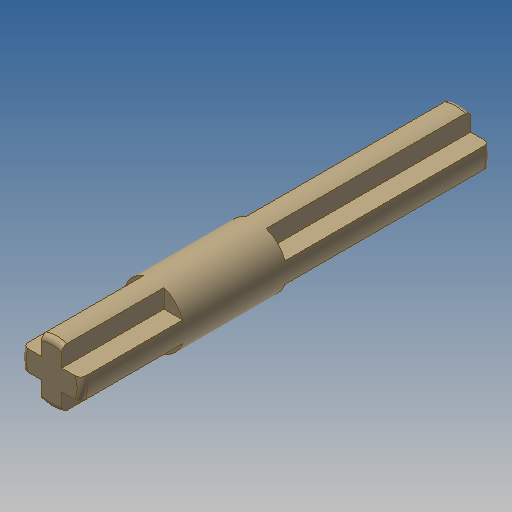
# Autodesk Inventor part: 99008-Tan
Saved by Autodesk Inventor 2022.2 (Build 262287000, 287)
## iProperties
Created: 2014-11-20
Part Number: 99008-Tan
Material: ABS Plastic
Document SubType Name: Modeling
Designer: D. Kohfeld
Mass: 0.471237 g
Surface Area: 5.91487 cm^2
Volume: 0.444563 cm^3
Density: 1.06 g/cm^3
Appearance: Tan
Author: D. Kohfeld
Autodesk Inventor part; units mm, degrees
ref_plane "YZ Plane" through (0, 0, 0) normal (1, 0, 0) x (0, 1, 0)
ref_plane "XZ Plane" through (0, 0, 0) normal (0, 1, 0) x (-1, 0, 0)
ref_plane "XY Plane" through (0, 0, 0) normal (0, 0, 1) x (1, 0, 0)
sketch "Sketch1" plane through (0, 0, 0) normal (0, 0, 1) x (1, 0, 0)
  circle A0 centre (0, 0) radius 2.4
  dimension "d0" = 4.8
  constraints: 1 centre point, 1 coincident
  measures "d0" diameter of A0
extrude "Extrusion1" add sketch "Sketch1" along normal mid plane 8
sketch "Sketch2" plane through (0, 0, 4) normal (0, 0, 1) x (1, 0, 0)
  circle A0 centre (0, 0) radius 2.4 projected
  line L0 (-0.8, 2.2627) -> (-0.8, 0.8)
  line L1 (-0.8, 0.8) -> (-2.2627, 0.8)
  line L2 (-2.2627, -0.8) -> (-0.8, -0.8)
  line L3 (-0.8, -0.8) -> (-0.8, -2.2627)
  line L4 (0.8, -2.2627) -> (0.8, -0.8)
  line L5 (0.8, -0.8) -> (2.2627, -0.8)
  line L6 (2.2627, 0.8) -> (0.8, 0.8)
  line L7 (0.8, 0.8) -> (0.8, 2.2627)
  dimension "d4" = 1.6
  constraints: 16 end point, 7 equal length, 4 perpendicular, 3 parallel, 1 vertical, 9 other
  measures "d4" distance between parallel lines of L7 L0
extrude "Extrusion2" add sketch "Sketch2" along normal blind 8 contours A0 L5 L4 L3 L2 L1 L0 L7 L6
sketch "Sketch3" plane through (0, 0, -4) normal (0, 0, -1) x (-1, 0, 0)
  circle A0 centre (0, 0) radius 2.4 projected
  line L0 (-0.8, 2.2627) -> (-0.8, 0.8)
  line L1 (-0.8, 0.8) -> (-2.2627, 0.8)
  line L2 (-2.2627, -0.8) -> (-0.8, -0.8)
  line L3 (-0.8, -0.8) -> (-0.8, -2.2627)
  line L4 (0.8, -2.2627) -> (0.8, -0.8)
  line L5 (0.8, -0.8) -> (2.2627, -0.8)
  line L6 (2.2627, 0.8) -> (0.8, 0.8)
  line L7 (0.8, 0.8) -> (0.8, 2.2627)
  dimension "d7" = 1.6
  constraints: 16 end point, 7 equal length, 4 perpendicular, 3 parallel, 1 vertical, 9 other
  measures "d7" distance between parallel lines of L0 L7
extrude "Extrusion3" add sketch "Sketch3" along normal blind 16 contours A0 L5 L4 L3 L2 L1 L0 L7 L6
fillet "Fillet1" radius 0.4 8 edges at (-2.4, 0, 12) (0, 2.4, 12) (2.4, 0, 12) (0, -2.4, 12) (0, -2.4, -20) (-2.4, 0, -20) (0, 2.4, -20) (2.4, 0, -20)
equation "\"d0\" = kd"
equation "\"d1\" = lu"
equation "\"d4\" = axlet"
equation "\"d5\" = lu"
equation "\"d7\" = axlet"
equation "\"d8\" = 2 * lu"
equation "\"d11\" = tf"
equation "\"kd\" = 4.8"
equation "\"lu\" = 8"
equation "\"axlet\" = 1.6"
equation "\"tf\" = 0.4"
body "Solid1"
